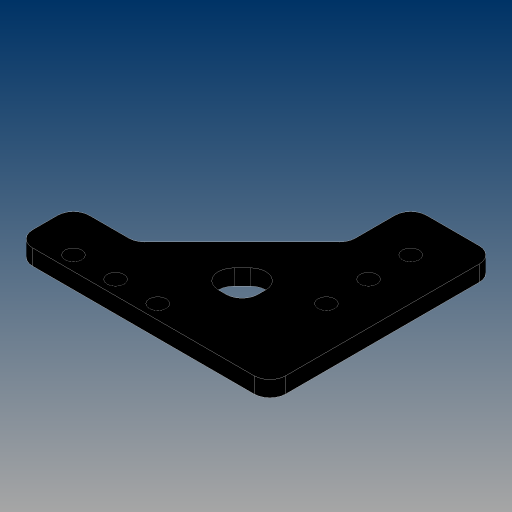
# Autodesk Inventor part: ELEV_007_SUPBRK2
Saved by Autodesk Inventor 2024.3 (Build 283343000, 343)
## iProperties
Created: 2024-11-25
Part Number: ELEV_007_SUPBRK2
Material: Aluminum 6061
Document SubType Name: Modeling
Designer: Kenji
Density: 2.7 g/cm^3
Appearance: Anodized - Black
Author: Kenji
Autodesk Inventor part; units mm, degrees
ref_plane "YZ Plane" through (0, 0, 0) normal (1, 0, 0) x (0, 1, 0)
ref_plane "XZ Plane" through (0, 0, 0) normal (0, 1, 0) x (-1, 0, 0)
ref_plane "XY Plane" through (0, 0, 0) normal (0, 0, 1) x (1, 0, 0)
sketch "Sketch1" plane through (0, 0, 0) normal (0, 1, 0) x (-1, 0, 0)
  line L0 (0, -11.8745) -> (0, -71.4375)
  line L1 (4.7625, -76.2) -> (20.6375, -76.2)
  line L2 (76.2, -20.6375) -> (76.2, -11.8745)
  line L3 (71.4375, -7.112) -> (4.7625, -7.112)
  circle A0 centre (12.7, -38.1) radius 2.54
  arc A1 (4.7625, -7.112) -> (0, -11.8745) centre (4.7625, -11.8745) ccw
  circle A2 centre (12.7, -50.8) radius 2.54
  circle A3 centre (12.7, -63.5) radius 2.54
  circle A4 centre (38.1, -12.7) radius 2.54
  circle A5 centre (50.8, -12.7) radius 2.54
  circle A6 centre (63.5, -12.7) radius 2.54
  line L4 (14.4961, -61.7039) -> (61.7039, -14.4961) construction
  line L5 (26.7949, -56.1403) -> (56.1403, -26.7949)
  line L6 (33.5301, -35.9347) -> (35.9347, -33.5301)
  line L7 (25.4, -76.2) -> (25.4, -25.4) construction
  line L8 (76.2, -25.4) -> (25.4, -25.4) construction
  line L9 (25.4, -59.5079) -> (25.4, -71.4375)
  line L10 (71.4375, -25.4) -> (59.5079, -25.4)
  arc A7 (71.4375, -25.4) -> (76.2, -20.6375) centre (71.4375, -20.6375) ccw
  arc A8 (76.2, -11.8745) -> (71.4375, -7.112) centre (71.4375, -11.8745) ccw
  arc A9 (20.6375, -76.2) -> (25.4, -71.4375) centre (20.6375, -71.4375) ccw
  arc A10 (0, -71.4375) -> (4.7625, -76.2) centre (4.7625, -71.4375) ccw
  line L11 (32.5671, -25.4) -> (30.1625, -25.4)
  line L12 (25.4, -32.5671) -> (25.4, -30.1625)
  arc A11 (59.5079, -25.4) -> (56.1403, -26.7949) centre (59.5079, -30.1625) ccw
  arc A12 (26.7949, -56.1403) -> (25.4, -59.5079) centre (30.1625, -59.5079) ccw
  arc A13 (35.9347, -33.5301) -> (32.5671, -25.4) centre (32.5671, -30.1625) ccw
  arc A14 (25.4, -32.5671) -> (33.5301, -35.9347) centre (30.1625, -32.5671) ccw
  arc A15 (30.1625, -25.4) -> (25.4, -30.1625) centre (30.1625, -30.1625) ccw
  point P0 (0, 0)
  point P1 (0, -76.2)
  point P2 (25.4, -57.5352)
  point P3 (57.5352, -25.4)
  point P4 (25.4, -44.0648)
  point P5 (44.0648, -25.4)
  dimension "d2" = 76.2
  dimension "d4" = 5.08
  dimension "d5" = 4.7625
  dimension "d7" = 12.7
  dimension "d8" = 12.7
  dimension "d9" = 12.7
  dimension "d10" = 5.08
  dimension "d11" = 12.7
  dimension "d12" = 12.7
  dimension "d13" = 38.1
  dimension "d18" = 25.4
  dimension "d20" = 4.7625
  dimension "d21" = 4.7625
  dimension "d22" = 4.7625
  dimension "d23" = 4.7625
  dimension "d24" = 4.7625
  dimension "d29" = 18.288
  dimension "d30" = 25.4
  dimension "d31" = 76.2
  dimension "d32" = 12.7
  dimension "d33" = 38.1
  constraints: 26 end point, 23 point on line, 20 point on circle, 20 tangent, 14 centre point, 7 equal radius, 3 perpendicular, 3 vertical, 2 horizontal, 2 horizontal alignment, 2 parallel, 2 vertical alignment, 1 collinear, 9 other
  measures "d2" distance between parallel lines of L0 L2
  measures "d4" diameter of A0
  measures "d5" radius of A1
  measures "d7" distance from line of L0 point (12.7, -63.5)
  measures "d8" distance of A2.centre A0.centre
  measures "d9" distance of point (12.7, -63.5) A2.centre
  measures "d10" diameter of A5
  measures "d11" distance of A4.centre A5.centre
  measures "d12" distance of A5.centre point (63.5, -12.7)
  measures "d13" distance from line of L0 A4.centre
  measures "d18" distance of point (0, -76.2) L7.start
  measures "d20" distance between parallel lines of L4 L5
  measures "d21" distance between parallel lines of L4 L6
  measures "d22" radius of A7
  measures "d23" radius of A9
  measures "d24" radius of A11
  measures "d29" distance between parallel lines of L3 L10
  measures "d30" distance from line of point (0, 0) L8
  measures "d31" distance from line of point (0, 0) L1
  measures "d32" vertical distance of point (0, 0) A4.centre
  measures "d33" vertical distance of point (0, 0) A0.centre
extrude "Extrusion1" add sketch "Sketch1" along normal blind 4.7625
sketch "Sketch2" plane through (0, 4.7625, 0) normal (0, 1, 0) x (1, 0, 0)
  line L0 (-71.4375, 7.112) -> (-4.7625, 7.112) projected
  line L1 (-76.2, 8.382) -> (0, 8.382)
  line L2 (-76.2, 20.6375) -> (-76.2, 11.8745) projected
  line L3 (0, 11.8745) -> (0, 71.4375) projected
  line L4 (-4.7625, 7.112) -> (0, 7.112)
  line L5 (0, 7.112) -> (0, 8.382)
  line L6 (-76.2, 8.382) -> (-76.2, 7.112)
  line L7 (-76.2, 7.112) -> (-71.4375, 7.112)
  point P0 (0, 0)
  dimension "d34" = 1.27
  constraints: 10 end point, 3 point on line, 2 parallel, 2 perpendicular, 1 horizontal
  measures "d34" distance between parallel lines of L0 L1
extrude "Extrusion2" cut sketch "Sketch2" against normal through all
fillet "Fillet1" radius 4.7752 2 edges at (-74.6754, 2.3813, -8.382) (-1.5246, 2.3813, -8.382)
body "Solid1"
